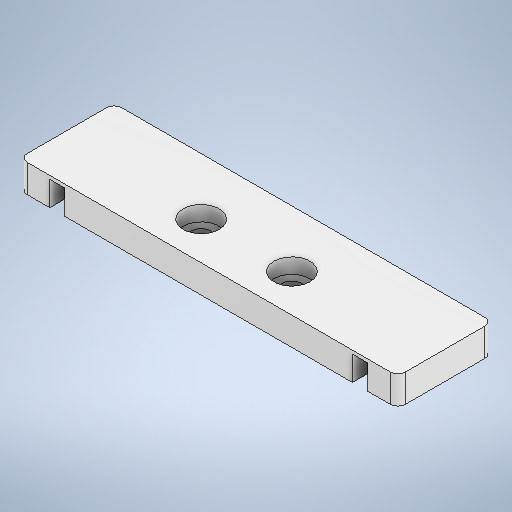
# Autodesk Inventor part: Limit Switch Bracket
Saved by Autodesk Inventor 2026.2 (Build 302298010, 298A)
## iProperties
Created: 2026-04-29
Part Number: Limit Switch Bracket
Material: ABS Plastic
Document SubType Name: Modeling
Designer: chanh
Density: 1.06 g/cm^3
Appearance: Smooth - White
Author: chanh
Autodesk Inventor part; units mm, degrees
ref_plane "YZ Plane" through (0, 0, 0) normal (1, 0, 0) x (0, 1, 0)
ref_plane "XZ Plane" through (0, 0, 0) normal (0, 1, 0) x (-1, 0, 0)
ref_plane "XY Plane" through (0, 0, 0) normal (0, 0, 1) x (1, 0, 0)
sketch "Sketch1" plane through (0, 0, 0) normal (0, 1, 0) x (-1, 0, 0)
  line L0 (50, -12.5) -> (-50, -12.5)
  line L1 (-50, -12.5) -> (-50, 12.5)
  line L2 (-50, 12.5) -> (50, 12.5)
  line L3 (50, 12.5) -> (50, -12.5)
  line L4 (50, -12.5) -> (-50, 12.5) construction
  line L5 (-50, -12.5) -> (50, 12.5) construction
  point P0 (0, 0)
  dimension "d0" = 100
  dimension "d1" = 25
  constraints: 12 end point, 2 midpoint, 2 parallel, 1 horizontal, 1 perpendicular
  measures "d0" distance of L1.end L2.end
  measures "d1" distance of L0.end L1.end
extrude "Extrusion1" add sketch "Sketch1" along normal blind 7.4
sketch "Sketch2" plane through (0, 7.4, 0) normal (0, 1, 0) x (1, 0, 0)
  line L0 (-32.5, 12.8309) -> (-37.5, 12.8309) projected
  line L1 (-37.5, 12.8309) -> (-37.5, 27.8309) projected
  line L2 (-37.5, 27.8309) -> (-32.5, 27.8309) projected
  line L3 (-32.5, 27.8309) -> (-32.5, 12.8309) projected
  line L4 (32.5, 12.8309) -> (37.5, 12.8309) projected
  line L5 (32.5, 27.8309) -> (32.5, 12.8309) projected
  line L6 (37.5, 27.8309) -> (32.5, 27.8309) projected
  line L7 (37.5, 12.8309) -> (37.5, 27.8309) projected
  line L8 (-50, -12.5) -> (50, -12.5) projected
  line L9 (50, -12.5) -> (50, 12.5) projected
  line L10 (50, 12.5) -> (-50, 12.5) projected
  line L11 (-50, 12.5) -> (-50, -12.5) projected
  line L12 (-42, 12.5) -> (-22, 12.5)
  line L13 (-22, 12.5) -> (-22, -3.5)
  line L14 (-22, -3.5) -> (-42, -3.5)
  line L15 (-42, -3.5) -> (-42, 12.5)
  line L16 (-42, -3.5) -> (-42, -12.5)
  line L17 (-38, -3.5) -> (-38, -12.5)
  point P0 (0, 0)
  point P1 (-35, 12.8309)
  point P2 (-22, 12.5)
  dimension "d4" = 7
  dimension "d5" = 20
  dimension "d6" = 16
  dimension "d7" = 4
  constraints: 12 end point, 4 point on line, 3 perpendicular, 2 parallel, 1 horizontal, 1 midpoint
  measures "d4" distance from line of L15 point (-35, 12.831)
  measures "d5" distance between parallel lines of L13 L15
  measures "d6" distance between parallel lines of L10 L14
  measures "d7" distance between parallel lines of L17 L16
sketch "Sketch3" plane through (0, 7.4, 0) normal (0, 1, 0) x (1, 0, 0)
  line L0 (50, 12.5) -> (-50, 12.5) projected
  line L1 (-50, -12.5) -> (50, -12.5) projected
  line L2 (50, -12.5) -> (50, 12.5) projected
  line L3 (-50, 12.5) -> (-50, -12.5) projected
  point P0 (0, 0)
  point P1 (12, -2.5)
  dimension "d11" = 12
  dimension "d12" = 15
  measures "d11" horizontal distance of point (12, -2.5) point (0, 0)
  measures "d12" distance from line of L0 point (12, -2.5)
hole "Hole1" at (12, 7.4, 2.5) direction (0, -1, 0) diameter 5.2 end through all counterbore diameter 9.5 counterbore depth 4
fillet "Fillet1" radius 2 4 edges at (50, 3.7, 12.5) (50, 3.7, -12.5) (-50, 3.7, 12.5) (-50, 3.7, -12.5)
sketch "Sketch4" plane through (0, 0, 0) normal (0, -1, 0) x (1, 0, 0)
  line L0 (-22, -12.5) -> (-22, 3.5) projected
  line L1 (-22, 3.5) -> (-42, 3.5) projected
  line L2 (48, -12.5) -> (-48, -12.5) projected
  line L3 (-42, 3.5) -> (-42, -12.5) projected
  line L4 (-42, 3.5) -> (-42, 12.5) projected
  line L5 (-38, 3.5) -> (-38, 12.5) projected
  line L6 (-48, 12.5) -> (48, 12.5) projected
  point P0 (0, 0)
extrude "Extrusion3" cut sketch "Sketch4" against normal blind 6.5
mirror "Mirror2" about plane through (0, 0, 0) normal (1, 0, 0) of "Hole1", "Extrusion3"
body "Solid1"
